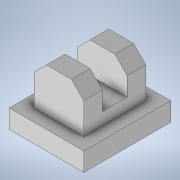
# Autodesk Inventor part: BT020_Doppelführung
Saved by Autodesk Inventor 2022 (Build 260153000, 153)
## iProperties
Created: 2022-01-06
Part Number: BT020_Doppelführung
Material: Generic
Document SubType Name: Modeling
Designer: Rayen
Density: 1 g/cm^3
Appearance: Default
Author: Rayen
Autodesk Inventor part; units mm, degrees
ref_plane "YZ Plane" through (0, 0, 0) normal (1, 0, 0) x (0, 1, 0)
sketch "Sketch1" plane through (0, 0, 0) normal (0, 0, 1) x (1, 0, 0)
  line L0 (-368.5938, -273.4375) -> (-368.5938, 352.1875)
  line L1 (-368.5938, 352.1875) -> (331.4062, 352.1875)
  line L2 (331.4062, 352.1875) -> (331.4062, -247.8125)
  line L3 (331.4062, -247.8125) -> (-368.5938, -247.8125)
  line L4 (-368.5938, -247.8125) -> (-368.5938, -273.4375)
  point P0 (0, 0)
  dimension "d0" = 700
  dimension "d1" = 600
  constraints: 10 end point, 4 perpendicular, 1 point on line, 1 vertical
  measures "d0" distance of L0.end L1.end
  measures "d1" distance of L1.end L2.end
extrude "Extrusion1" add sketch "Sketch1" along normal blind 150
ref_plane "Work Plane1" through (0, 0, 150) normal (0, 0, 1) x (1, 0, 0)
sketch "Sketch2" plane through (0, 0, 150) normal (0, 0, 1) x (1, 0, 0)
  line L0 (-268.5938, -147.8125) -> (-268.5938, 252.1875)
  line L1 (-268.5938, 252.1875) -> (231.4062, 252.1875)
  line L2 (231.4062, 252.1875) -> (231.4063, -147.8125)
  line L3 (231.4063, -147.8125) -> (-268.5938, -147.8125)
  line L4 (331.4062, 352.1875) -> (-368.5938, 352.1875) projected
  line L5 (331.4062, -247.8125) -> (331.4062, 352.1875) projected
  point P0 (0, 0)
  dimension "d5" = 500
  dimension "d6" = 400
  dimension "d7" = 100
  dimension "d8" = 100
  constraints: 8 end point, 3 perpendicular, 1 vertical
  measures "d5" distance of L0.end L1.end
  measures "d6" distance of L0.start L0.end
  measures "d7" distance between parallel lines of L4 L1
  measures "d8" distance between parallel lines of L5 L2
extrude "Extrusion2" add sketch "Sketch2" along normal blind 100
sketch "Sketch3" plane through (231.4062, -147.8125, 150) normal (1, 0, 0) x (0, 0, -1)
  line L0 (-100, 0) -> (-100, 400) projected
  line L1 (-100, 0) -> (-250, 0)
  line L2 (-350, 100) -> (-350, 300)
  line L3 (-250, 400) -> (-100, 400)
  line L4 (0, 400) -> (-100, 400) projected
  line L5 (-250, 400) -> (-350, 300)
  line L6 (-250, 0) -> (-350, 100)
  point P0 (150, 147.8125)
  point P1 (-350, 0)
  point P2 (-350, 400)
  dimension "d11" = 250
  dimension "d12" = 400
  dimension "d13" = 100
  dimension "d14" = 45
  dimension "d15" = 100
  dimension "d16" = 45
  constraints: 10 end point, 6 point on line, 3 perpendicular, 1 collinear
  measures "d11" distance of point (-350, 400) L3.end
  measures "d12" distance of point (-350, 0) point (-350, 400)
  measures "d13" distance of L3.start point (-350, 400)
  measures "d14" angle of L3 L5
  measures "d15" distance of L1.end point (-350, 0)
  measures "d16" angle of L1 L6
extrude "Extrusion3" add sketch "Sketch3" against normal blind 150
ref_plane "Work Plane2" through (-18.5938, -147.8125, 150) normal (1, 0, 0) x (0, 0, -1)
mirror "Mirror1" about plane through (-18.5938, -147.8125, 150) normal (1, 0, 0) of "Extrusion3"
equation "\"d15\" = d13"
equation "\"d16\" = d14"
body "Solid1"
